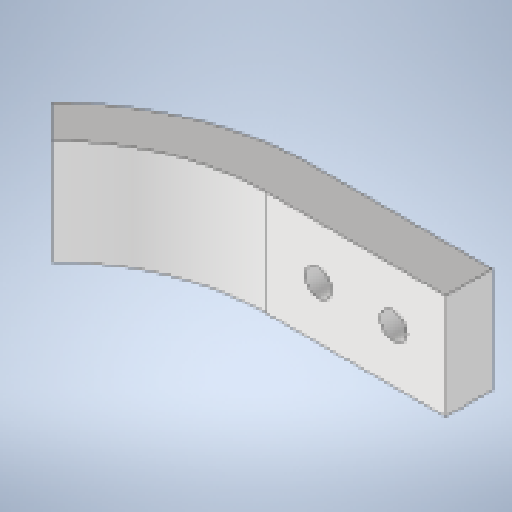
# Autodesk Inventor part: KickerFoot
Saved by Autodesk Inventor 2025.1 (Build 291241000, 241)
## iProperties
Created: 2026-04-18
Part Number: KickerFoot
Material: Generic
Document SubType Name: Modeling
Designer: User
Density: 1 g/cm^3
Appearance: Default
Author: User
## iProperties of the stored document KickerFoot_3DPrint.ipt
Created: 2026-04-18
Part Number: KickerFoot_3DPrint
Material: Generic
Document SubType Name: Modeling
Designer: User
Density: 1 g/cm^3
Appearance: Default
Author: User
Autodesk Inventor part; units mm, degrees
ref_plane "YZ Plane" through (0, 0, 0) normal (1, 0, 0) x (0, 1, 0)
ref_plane "XZ Plane" through (0, 0, 0) normal (0, 1, 0) x (-1, 0, 0)
sketch "Sketch1" plane through (0, 0, 0) normal (0, 0, 1) x (1, 0, 0)
  circle A0 centre (-4.048211, 0) radius 1.45
  circle A1 centre (4.048211, 0) radius 1.45
  line L0 (-8, 3.951789) -> (-8, -3.951789)
  line L1 (-8, -3.951789) -> (8, -3.951789)
  line L2 (8, -3.951789) -> (8, 3.951789)
  line L3 (8, 3.951789) -> (-8, 3.951789)
  line L4 (8.2, 4.151789) -> (8.2, -4.151789)
  line L5 (8.2, -4.151789) -> (-8.2, -4.151789)
  line L6 (-8.2, -4.151789) -> (-8.2, 4.151789)
  line L7 (-8.2, 4.151789) -> (8.2, 4.151789)
  point P0 (0, 0)
  dimension "d0" = 0.2
  constraints: 8 end point, 3 other
  measures "d0" distance between parallel lines of L2 L4
sketch "Sketch1 outline for Extrusion1" plane through (0, 0, 0) normal (0, 0, 1) x (1, 0, 0)
  line L0 (8.2, 4.151789) -> (-8.2, 4.151789)
  line L1 (8.2, -4.151789) -> (8.2, 4.151789)
  line L2 (-8.2, 4.151789) -> (-8.2, -4.151789)
  line L3 (-8.2, -4.151789) -> (8.2, -4.151789)
  circle A0 centre (4.048211, 0) radius 1.45
  circle A1 centre (-4.048211, 0) radius 1.45
extrude "Extrusion1" add sketch "Sketch1 outline for Extrusion1" along normal blind 2
sketch "Sketch2" plane through (0, 0, 2) normal (0, 0, 1) x (1, 0, 0)
  line L0 (8.2, -4.151789) -> (8.2, 4.151789)
  line L1 (8.2, 4.151789) -> (-8.2, 4.151789)
  line L2 (-8.2, 4.151789) -> (-8.2, -4.151789)
  line L3 (-8.2, -4.151789) -> (8.2, -4.151789)
  line L4 (9.7, 5.651789) -> (9.7, -5.651789)
  line L5 (9.7, -5.651789) -> (-9.7, -5.651789)
  line L6 (-9.7, -5.651789) -> (-9.7, 5.651789)
  line L7 (-9.7, 5.651789) -> (9.7, 5.651789)
  point P0 (0, 0)
  dimension "d3" = 1.5
  constraints: 8 end point, 3 other
  measures "d3" distance between parallel lines of L0 L4
ref_plane "Work Plane1" through (7.997687, -5.958328, -3) normal (0, 0, 1) x (1, 0, 0)
sketch "Sketch2 outline for Extrusion2" plane through (0, 0, 2) normal (0, 0, 1) x (1, 0, 0)
  line L0 (9.7, 5.651789) -> (-9.7, 5.651789)
  line L1 (9.7, -5.651789) -> (9.7, 5.651789)
  line L2 (-9.7, 5.651789) -> (-9.7, -5.651789)
  line L3 (-9.7, -5.651789) -> (9.7, -5.651789)
  line L4 (8.2, -4.151789) -> (-8.2, -4.151789)
  line L5 (8.2, 4.151789) -> (8.2, -4.151789)
  line L6 (-8.2, 4.151789) -> (8.2, 4.151789)
  line L7 (-8.2, -4.151789) -> (-8.2, 4.151789)
extrude "Extrusion2" add sketch "Sketch2 outline for Extrusion2" against normal up to surface (5 mm away)
sketch "Sketch3" plane through (-9.7, 5.651789, 2) normal (0, 1, 0) x (1, 0, 0)
  line L0 (0, 0) -> (0, 5)
  line L1 (0, 0) -> (0, -23)
  line L2 (0, -23) -> (-19.79899, -3.20101)
  line L3 (0, -23) -> (28, -23) construction
  arc A0 (-33.20486, -51.037646) -> (-33.20486, -51.037646) centre (1.795137, -51.024043) ccw
  arc A1 (-33.20486, -51.037646) -> (-33.20486, -51.037646) centre (1.795137, -51.024043) ccw
  line L4 (0, -23) -> (0, -58)
  line L5 (0, -58) -> (2, -58)
  arc A2 (-26.992777, -30.442444) -> (-24.224883, -27.796432) centre (2, -58) ccw
  line L6 (-24.218855, -43.305973) -> (-24.238811, 8.039757)
  line L7 (19.4, 0) -> (19.4, 5)
  line L8 (19.4, 5) -> (19.4, -23)
  line L9 (2, -23) -> (19.4, -23)
  line L10 (0, 0) -> (19.4, 0)
  arc A3 (-24.221288, -37.047392) -> (28, -23) centre (0, -23) ccw
  arc A4 (0, -46) -> (23, -23) centre (0, -23) ccw
  arc A5 (-26.992777, -30.442444) -> (-24.962512, -35.683572) centre (0, -23) ccw
  arc A6 (2, -23) -> (-24.222154, -34.81814) centre (2, -58) ccw
  arc A7 (-24.962512, -35.683572) -> (22.105735, -29.351101) centre (2, -58) ccw
  arc A8 (0, 5) -> (-24.2322, -8.97144) centre (0, -23) ccw
  arc A9 (19.4, -10.645244) -> (0, 0) centre (0, -23) ccw
  point P0 (9.7, 2)
  point P1 (0, -23)
  point P2 (0, -23)
  point P3 (0, -23.05719)
  dimension "d6" = 23
  dimension "d7" = 135
  dimension "d21" = 35
  dimension "d23" = 2
  constraints: 18 point on circle, 15 end point, 8 centre point, 8 point on line, 4 coincident, 2 perpendicular, 2 vertical, 1 equal length, 1 horizontal, 10 other
  measures "d6" distance of L0.start L1.end
  measures "d7" angle of L3 L2
  measures "d21" distance of L2.start L4.end
  measures "d23" distance of L5.start L5.end
sketch "Sketch3 outline for Extrusion3" plane through (-9.7, 5.651789, 2) normal (0, 1, 0) x (1, 0, 0)
  line L0 (19.4, 0) -> (0, 0)
  line L1 (0, 0) -> (0, 5)
  arc A0 (0, 5) -> (-24.2322, -8.97144) centre (0, -23) ccw
  line L2 (-24.2322, -8.97144) -> (-24.222154, -34.81814)
  arc A1 (-24.222154, -34.81814) -> (2, -23) centre (2, -58) cw
  line L3 (2, -23) -> (19.4, -23)
  line L4 (19.4, -23) -> (19.4, 0)
extrude "Extrusion3" add sketch "Sketch3 outline for Extrusion3" against normal up to surface (11.303579 mm away)
sketch "Sketch18" plane through (-7.7, 5.651789, 25) normal (0, 1, 0) x (1, 0, 0)
  line L0 (-2, 28) -> (17.4, 28)
  arc A0 (-2, 28) -> (-26.2322, 14.02856) centre (-2, 0) ccw
  line L1 (-26.2322, 14.02856) -> (-26.222154, -11.81814)
  arc A1 (0, 0) -> (-26.222154, -11.81814) centre (0, -35) ccw
  line L2 (0, 0) -> (17.4, 0)
  line L3 (17.4, 0) -> (17.4, 28)
  point P0 (7.7, 25)
sketch "Sketch18 outline for Extrusion15" plane through (-7.7, 5.651789, 25) normal (0, 1, 0) x (1, 0, 0)
  line L0 (-26.2322, 14.02856) -> (-26.222154, -11.81814)
  arc A0 (-2, 28) -> (-26.2322, 14.02856) centre (-2, 0) ccw
  line L1 (17.4, 28) -> (-2, 28)
  line L2 (17.4, 0) -> (17.4, 28)
  line L3 (0, 0) -> (17.4, 0)
  arc A1 (-26.222154, -11.81814) -> (0, 0) centre (0, -35) cw
extrude "Extrusion15" add sketch "Sketch18 outline for Extrusion15" along normal blind 47.75
sketch "Sketch19" plane through (-9.7, -5.651789, -3) normal (0, -1, 0) x (1, 0, 0)
  line L0 (19.4, 0) -> (0, 0)
  line L1 (19.4, 28) -> (19.4, 0)
  line L2 (2, 28) -> (19.4, 28)
  arc A0 (-24.222154, 39.81814) -> (2, 28) centre (2, 63) ccw
  line L3 (-24.2322, 13.97144) -> (-24.222154, 39.81814)
  arc A1 (-24.2322, 13.97144) -> (0, 0) centre (0, 28) ccw
  point P0 (9.7, 3)
sketch "Sketch19 outline for Extrusion16" plane through (-9.7, -5.651789, -3) normal (0, -1, 0) x (1, 0, 0)
  arc A0 (-24.2322, 13.97144) -> (0, 0) centre (0, 28) ccw
  line L0 (-24.222154, 39.81814) -> (-24.2322, 13.97144)
  arc A1 (2, 28) -> (-24.222154, 39.81814) centre (2, 63) cw
  line L1 (19.4, 28) -> (2, 28)
  line L2 (19.4, 0) -> (19.4, 28)
  line L3 (0, 0) -> (19.4, 0)
extrude "Extrusion16" add sketch "Sketch19 outline for Extrusion16" along normal blind 47.75
sketch "Sketch20" plane through (9.7, 53.401789, 25) normal (1, 0, 0) x (0, 0, -1)
  circle A0 centre (-28.024043, -53.730658) radius 35
  line L0 (0, 0) -> (0, -106.803579)
  line L1 (-28.024043, -53.730658) -> (0, -54.184091)
  line L2 (0, -54.184091) -> (6.97302, -54.184091)
  line L3 (0, -54.184091) -> (6.97302, -54.184091) construction
  line L4 (0, -106.803579) -> (0, 0)
  line L5 (-11.81814, 0) -> (0, 0)
  line L6 (-11.81814, -106.803579) -> (-11.81814, 0)
  line L7 (0, -106.803579) -> (-11.81814, -106.803579)
  circle A1 centre (-28.024043, -53.730658) radius 40
  arc A2 (0, -54.184091) -> (-11.81814, -17.160606) centre (-61.997018, -53.575991) ccw
  arc A3 (-11.81814, -90.30071) -> (0, -54.184091) centre (-61.999295, -53.888464) ccw
  point P0 (25, -53.401789)
  point P1 (0, -52.967891)
  dimension "d55" = 0
  dimension "d56" = 6.97302
  dimension "d57" = 5
  dimension "d58" = 62
  dimension "d59" = 62
  constraints: 6 end point, 6 point on circle, 3 centre point, 3 point on line, 1 collinear, 1 horizontal, 4 other
  measures "d55" distance between parallel lines of L2 L3
  measures "d56" distance of L1.end L2.end
  measures "d58" radius of A2
  measures "d59" radius of A3
sketch "Sketch20 outline for Extrusion17" plane through (9.7, 53.401789, 25) normal (1, 0, 0) x (0, 0, -1)
  arc A0 (0, -54.184091) -> (-11.81814, -90.30071) centre (-61.999295, -53.888464) cw
  line L0 (0, -106.803579) -> (0, -54.184091)
  line L1 (-11.81814, -106.803579) -> (0, -106.803579)
  line L2 (-11.81814, -90.30071) -> (-11.81814, -106.803579)
  arc A1 (-11.81814, -17.160606) -> (0, -52.967891) centre (-61.997018, -53.575991) cw
  line L3 (-11.81814, 0) -> (-11.81814, -17.160606)
  line L4 (0, 0) -> (-11.81814, 0)
  line L5 (0, -52.967891) -> (0, 0)
  arc A2 (0, -54.184091) -> (0, -52.967891) centre (-61.997018, -53.575991) ccw
  line L6 (0, -52.967891) -> (0, -54.184091)
extrude "Extrusion17" add sketch "Sketch20 outline for Extrusion17" against normal up to surface (43.626747 mm away)
sketch "Sketch21" plane through (9.7, -53.401789, -3) normal (1, 0, 0) x (0, 0, -1)
  line L0 (-48.305973, 110.199312) -> (3.039757, 58.853579)
  line L1 (3.015448, 47.95) -> (-48.305973, -3.371424)
  line L2 (-49.720186, 108.785098) -> (1.625543, 57.439365)
  line L3 (1.601234, 49.364214) -> (-49.720186, -1.957211)
  line L4 (0, 0) -> (-39.81814, 0)
  line L5 (0, 106.803579) -> (0, 0)
  line L6 (0, 106.803579) -> (-39.81814, 106.803579)
  line L7 (-39.81814, 106.803579) -> (-39.81814, 89.642972)
  arc A0 (-28, 53.835688) -> (-39.81814, 89.642972) centre (-89.997018, 53.227588) ccw
  line L8 (-28, 53.835688) -> (-28, 52.619488)
  arc A1 (-39.81814, 16.502868) -> (-28, 52.619488) centre (-89.999295, 52.915114) ccw
  line L9 (-39.81814, 16.502868) -> (-39.81814, 0)
  point P0 (-3, 53.401789)
  point P1 (0, 47.762979)
  point P2 (-39.81814, 7.944836)
  point P3 (-39.81814, 98.883051)
  point P4 (0, 59.064908)
  dimension "d62" = 2
  dimension "d63" = 2
  constraints: 4 end point, 2 parallel
  measures "d62" distance between parallel lines of L0 L2
  measures "d63" distance between parallel lines of L1 L3
sketch "Sketch21 outline for Extrusion18" plane through (9.7, -53.401789, -3) normal (1, 0, 0) x (0, 0, -1)
  line L0 (-39.81814, 0) -> (0, 0)
  line L1 (-39.81814, 7.944836) -> (-39.81814, 0)
  line L2 (0, 47.762979) -> (-39.81814, 7.944836)
  line L3 (0, 0) -> (0, 47.762979)
  line L4 (0, 106.803579) -> (-39.81814, 106.803579)
  line L5 (0, 59.064908) -> (0, 106.803579)
  line L6 (-39.81814, 98.883051) -> (0, 59.064908)
  line L7 (-39.81814, 106.803579) -> (-39.81814, 98.883051)
extrude "Extrusion18" cut sketch "Sketch21 outline for Extrusion18" against normal through all
fillet "Fillet2" radius 40 2 edges at (-12.1111, -36.8989, 36.8181) (-12.1111, 36.2412, 36.8181)
sketch "Sketch22" plane through (9.7, -5.63881, -3) normal (1, 0, 0) x (0, 0, -1)
  line L0 (0, -0.312979) -> (0, 11.590599)
  line L1 (-39.81814, -39.818143) -> (0, 0)
  line L2 (0, 11.301929) -> (-39.81814, 51.120072)
  arc A0 (-28, 6.072708) -> (-35.216358, 34.500437) centre (-89.997018, 5.464608) ccw
  arc A1 (-35.246627, -23.936442) -> (-28, 4.856508) centre (-89.999295, 5.152135) ccw
  line L3 (-28, 6.072708) -> (-28, 4.856508)
  arc A2 (-35.246627, -23.936442) -> (-39.81814, -39.818143) centre (0.077675, -42.703266) ccw
  arc A3 (-39.81814, 51.120072) -> (-35.216358, 34.500437) centre (0.126003, 53.233229) ccw
  line L4 (-3.181981, 8.119949) -> (-30.774323, 35.712293)
  arc A4 (-23.5, 6.094391) -> (-30.774323, 35.712293) centre (-89.997018, 5.464608) ccw
  line L5 (-23.5, 6.094391) -> (-23.5, 4.845968)
  arc A5 (-30.103262, -23.739303) -> (-23.5, 4.845968) centre (-89.999295, 5.152135) ccw
  line L6 (-30.103262, -23.739303) -> (-3.181981, 3.18198)
  line L7 (-3, 9.590599) -> (-3, 1.687021)
  line L8 (-6, 9.590599) -> (-6, 1.687021)
  line L9 (0, 11.301929) -> (8.286805, 11.301929) construction
  line L10 (0, 11.301929) -> (-23.784266, 11.301929)
  line L11 (0, 11.301929) -> (23.784266, 11.301929) construction
  line L12 (0, 0) -> (-23.699178, 0)
  line L13 (0, 0) -> (23.699178, 0) construction
  line L14 (-30.103262, -23.739303) -> (-30.103262, -30.103264)
  line L15 (-30.774323, 35.712293) -> (-30.774323, 42.076254)
  point P0 (-3, 5.63881)
  point P1 (-23.699178, 0)
  point P2 (-23.753711, 11.301929)
  dimension "d67" = 4.5
  dimension "d68" = 3
  dimension "d70" = 180
  dimension "d71" = 180
  constraints: 22 end point, 5 point on circle, 3 horizontal, 2 centre point, 2 collinear, 2 parallel, 2 point on line, 1 vertical, 4 other
  measures "d67" distance between parallel lines of L2 L4
  measures "d68" distance between parallel lines of L7 L8
  measures "d70" angle of L10 L11
  measures "d71" angle of L12 L13
sketch "Sketch22 outline for Extrusion19" plane through (9.7, -5.63881, -3) normal (1, 0, 0) x (0, 0, -1)
  line L0 (0, 0) -> (-23.699178, 0)
  line L1 (-30.103262, -30.103264) -> (0, 0)
  line L2 (-30.103262, -23.739303) -> (-30.103262, -30.103264)
  arc A0 (-23.699178, 0) -> (-30.103262, -23.739303) centre (-89.999295, 5.152135) cw
  line L3 (-23.753711, 11.301929) -> (0, 11.301929)
  arc A1 (-30.774323, 35.712293) -> (-23.753711, 11.301929) centre (-89.997018, 5.464608) cw
  line L4 (-30.774323, 42.076254) -> (-30.774323, 35.712293)
  line L5 (0, 11.301929) -> (-30.774323, 42.076254)
extrude "Extrusion19" cut sketch "Sketch22 outline for Extrusion19" against normal through all
sketch "Sketch23" plane through (-7.7, -0.782301, 25) normal (0, 0, 1) x (1, 0, 0)
  line L0 (17.4, -4.856508) -> (-2, -4.856508)
  line L1 (-2, -4.856508) -> (-2, 6.44542)
  line L2 (-2, 6.44542) -> (17.4, 6.44542)
  line L3 (17.4, 6.44542) -> (17.4, -4.856508)
  line L4 (-0.5, 4.934091) -> (-0.5, -3.369488)
  line L5 (-0.5, -3.369488) -> (15.9, -3.369488)
  line L6 (15.9, -3.369488) -> (15.9, 4.934091)
  line L7 (15.9, 4.934091) -> (-0.5, 4.934091)
  point P0 (7.7, 0.782301)
sketch "Sketch23 outline for Extrusion20" plane through (-7.7, -0.782301, 25) normal (0, 0, 1) x (1, 0, 0)
  line L0 (-0.5, 4.934091) -> (-0.5, -3.369488)
  line L1 (15.9, 4.934091) -> (-0.5, 4.934091)
  line L2 (15.9, -3.369488) -> (15.9, 4.934091)
  line L3 (-0.5, -3.369488) -> (15.9, -3.369488)
extrude "Extrusion20" cut sketch "Sketch23 outline for Extrusion20" against normal blind 22
sketch "Sketch26" plane through (9.7, -0.782301, 25) normal (0, 0, 1) x (1, 0, 0)
  line L0 (0, -4.856508) -> (-19.4, -4.856508)
  line L1 (-19.4, -4.856508) -> (-19.4, 6.44542)
  line L2 (-19.4, 6.44542) -> (0, 6.44542)
  line L3 (0, 6.44542) -> (0, -4.856508)
  line L4 (-17.9, 4.934091) -> (-17.9, -3.369488)
  line L5 (-17.9, -3.369488) -> (-1.5, -3.369488)
  line L6 (-1.5, -3.369488) -> (-1.5, 4.934091)
  line L7 (-1.5, 4.934091) -> (-17.9, 4.934091)
  point P0 (-9.7, 0.782301)
sketch "Sketch26 outline for Extrusion21" plane through (9.7, -0.782301, 25) normal (0, 0, 1) x (1, 0, 0)
  line L0 (-17.9, 4.934091) -> (-17.9, -3.369488)
  line L1 (-1.5, 4.934091) -> (-17.9, 4.934091)
  line L2 (-1.5, -3.369488) -> (-1.5, 4.934091)
  line L3 (-17.9, -3.369488) -> (-1.5, -3.369488)
extrude "Extrusion21" cut sketch "Sketch26 outline for Extrusion21" along normal blind 22
sketch "Sketch27" plane through (9.7, -5.63881, -3) normal (0, 0, -1) x (-1, 0, 0)
  circle A0 centre (5.651789, 5.63881) radius 1.45
  circle A1 centre (13.748211, 5.63881) radius 1.45
  point P0 (9.7, 5.63881)
sketch "Sketch27 outline for Extrusion22" plane through (9.7, -5.63881, -3) normal (0, 0, -1) x (-1, 0, 0)
  circle A0 centre (5.651789, 5.63881) radius 1.45
  circle A1 centre (13.748211, 5.63881) radius 1.45
extrude "Extrusion22" cut sketch "Sketch27 outline for Extrusion22" against normal blind 22
fillet "Fillet3" radius 10 2 edges at (-12.1142, 5.6631, 20.7537) (-12.1142, -5.6388, 20.6992)
body "Solid1"
